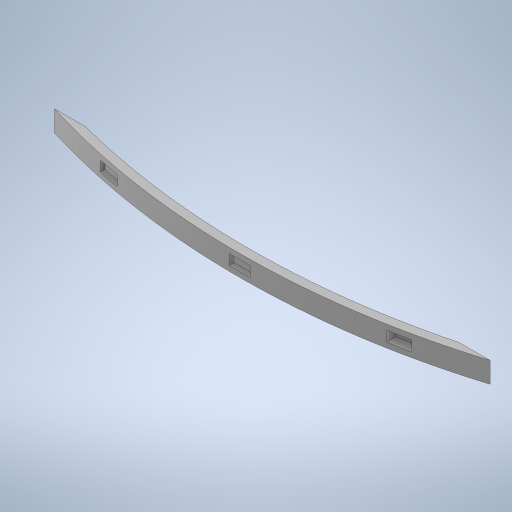
# Autodesk Inventor part: front_back band
Saved by Autodesk Inventor 2024 (Build 280153000, 153)
## iProperties
Created: 2025-11-15
Part Number: front_back band
Material: PC/ABS Plastic
Document SubType Name: Modeling
Designer: garys
Density: 1.1 g/cm^3
Appearance: Smooth - White
Author: garys
Autodesk Inventor part; units mm, degrees
ref_plane "YZ Plane" through (0, 0, 0) normal (1, 0, 0) x (0, 1, 0)
ref_plane "XZ Plane" through (0, 0, 0) normal (0, 1, 0) x (-1, 0, 0)
ref_plane "XY Plane" through (0, 0, 0) normal (0, 0, 1) x (1, 0, 0)
sketch "Sketch1" plane through (0, 0, 0) normal (0, 1, 0) x (-1, 0, 0)
  line L0 (0, 0) -> (114.3, 0)
  line L1 (0, 0) -> (-114.3, 0)
  arc A0 (114.3, 0) -> (-114.3, 0) centre (0, -439.988) ccw
  line L2 (114.3, 0) -> (133.35, 0)
  line L3 (-114.3, 0) -> (-133.35, 0)
  arc A1 (133.35, 0) -> (-133.35, 0) centre (0, -434.5851) ccw
  point P0 (0, 19.9987)
  point P1 (0, 14.604)
  dimension "d0" = 114.3
  dimension "d1" = 114.3
  dimension "d2" = 19.05
  dimension "d3" = 19.05
  dimension "d5" = 454.592
  dimension "d6" = 454.5838
  constraints: 8 end point, 6 point on circle, 4 horizontal, 2 centre point
  measures "d0" distance of L0.start L0.end
  measures "d1" distance of L0.start L1.end
  measures "d2" distance of L0.end L2.end
  measures "d3" distance of L1.end L3.end
  measures "d5" radius of A0
  measures "d6" radius of A1
extrude "Extrusion1" add sketch "Sketch1" along normal blind 12.7 contours A0 L3 A1 L2
sketch "Sketch2" plane through (133.35, 0, 0) normal (0, 0, -1) x (-1, 0, 0)
  line L0 (266.7, 12.7) -> (0, 12.7) projected
  line L1 (127, 9.525) -> (139.7, 9.525)
  line L2 (139.7, 9.525) -> (139.7, 3.175)
  line L3 (139.7, 3.175) -> (127, 3.175)
  line L4 (127, 3.175) -> (127, 9.525)
  line L5 (266.7, 0) -> (266.7, 12.7) projected
  line L6 (177.7987, 12.7) -> (177.7987, -0.436)
  line L7 (228.5974, 9.525) -> (215.8974, 9.525)
  line L8 (215.8974, 9.525) -> (215.8974, 3.175)
  line L9 (215.8974, 3.175) -> (228.5974, 3.175)
  line L10 (228.5974, 3.175) -> (228.5974, 9.525)
  line L11 (88.9, 12.7) -> (88.9, -0.436)
  line L12 (50.8, 9.525) -> (38.1, 9.525)
  line L13 (38.1, 9.525) -> (38.1, 3.175)
  line L14 (38.1, 3.175) -> (50.8, 3.175)
  line L15 (50.8, 3.175) -> (50.8, 9.525)
  point P0 (133.35, 0)
  point P1 (177.8, 6.35)
  point P2 (88.9, 6.35)
  dimension "d12" = 12.7
  dimension "d13" = 6.35
  dimension "d14" = 127
  dimension "d15" = 38.1
  dimension "d16" = 38.1
  constraints: 28 end point, 8 symmetric about line, 2 parallel, 2 point on line, 2 vertical, 1 horizontal, 1 perpendicular
  measures "d12" distance of L2.end L3.end
  measures "d13" distance of L1.end L2.end
  measures "d14" distance between parallel lines of L5 L2
  measures "d15" distance from line of L2 point (177.8, 6.35)
  measures "d16" distance from line of point (88.9, 6.35) L4
extrude "Extrusion2" cut sketch "Sketch2" against normal through all
sketch "Sketch4" plane through (82.55, 3.175, 12.4405) normal (0, 1, 0) x (1, 0, 0)
  line L0 (0, 5.3945) -> (0, 0) projected
  line L1 (0, 5.3945) -> (0, 2.7021)
  arc A0 (0, 5.3945) -> (12.7, 7.9273) centre (-82.55, 452.4285) ccw projected
  line L2 (12.7, 7.9273) -> (12.7, 5.2349)
  arc A1 (12.7, 7.9273) -> (0, 5.3945) centre (84.4999, -385.2031) ccw
  arc A2 (0, 2.7021) -> (12.7, 5.2349) centre (-40.4319, 238.5449) ccw
  point P0 (-82.55, 12.4405)
  dimension "d19" = 2.6924
  dimension "d20" = 2.6924
  constraints: 4 end point, 4 point on circle, 2 centre point, 1 point on line, 1 vertical
  measures "d19" distance of L0.start L1.end
  measures "d20" distance of L2.start L2.end
extrude "Extrusion3" add sketch "Sketch4" along normal blind 6.35 contours A1 A0
sketch "Sketch5" plane through (0, 3.175, -434.5851) normal (0, 1, 0) x (1, 0, 0)
  line L0 (6.35, -449.1448) -> (6.35, -451.8372)
  arc A0 (-114.3, -434.5851) -> (114.3, -434.5851) centre (0, 5.4029) ccw projected
  line L1 (-6.35, -449.1448) -> (-6.35, -451.8372)
  arc A1 (-6.35, -451.8372) -> (6.35, -451.8372) centre (0, -227.9789) ccw
  point P0 (0, -434.5851)
  dimension "d23" = 2.6924
  dimension "d24" = 2.6924
  constraints: 4 end point, 3 point on circle, 2 vertical, 1 centre point
  measures "d23" distance of L0.start L0.end
  measures "d24" distance of L1.start L1.end
extrude "Extrusion4" add sketch "Sketch5" along normal blind 6.35
sketch "Sketch6" plane through (-82.5474, 3.175, 12.441) normal (0, 1, 0) x (1, 0, 0)
  arc A0 (-12.7, 7.9272) -> (0, 5.3945) centre (82.5474, 452.429) ccw projected
  line L0 (0, 5.3945) -> (0, 2.7021)
  line L1 (0, 5.3945) -> (0, 0) projected
  line L2 (-12.7, 7.9272) -> (-12.7, 5.2348)
  line L3 (-12.7, 7.9272) -> (-12.7, 2.5327) projected
  arc A1 (-12.7, 7.9272) -> (0, 5.3945) centre (1241.181, 6262.2948) ccw
  arc A2 (-12.7, 5.2348) -> (0, 2.7021) centre (38.067, 226.6937) ccw
  point P0 (82.5474, 12.441)
  dimension "d27" = 2.6924
  dimension "d28" = 2.6924
  constraints: 4 end point, 4 point on circle, 2 centre point, 2 point on line
  measures "d27" distance of L0.start L0.end
  measures "d28" distance of L2.start L2.end
extrude "Extrusion5" add sketch "Sketch6" along normal blind 6.35
body "Solid1"
